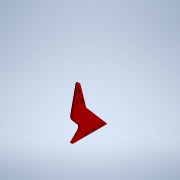
# Autodesk Inventor part: WeaponMountBasePlateV2
Saved by Autodesk Inventor 2020 (Build 240168000, 168)
## iProperties
Created: 2024-02-06
Part Number: WeaponMountBasePlateV2
Material: PETG
Document SubType Name: Modeling
Designer: smz3rm
Density: 1 g/cm^3
Appearance: Generic
Mass: 9.49681 g
Surface Area: 76.5782 cm^2
Volume: 9.49681 cm^3
WeaponHeight: 50.450 mm
SlotWidth: 6.000 mm
WeaponBite: 30.000 mm
WeaponMotorDia: 27.800 mm
SlotSpacing: 16.333 mm
SlotOffset: 2.000 mm
SlotHeight: 4.000 mm
SlotTolerance: 0.800 mm
WeaponMountBaseThinThickness: 1.000 mm
Height: 30.000 mm
BaseThickness: 3.000 mm
SideThickness: 6.000 mm
TopThickness: 1.000 mm
M3ScrewInsertBrim: 8.000 mm
M3ScrewDia: 3.100 mm
M3ScrewInsertDia: 4.000 mm
VM3ScrewInsertDia: 3.750 mm
FrontAngle: 45.00 deg
WeaponOpeningWidth: 15.000 mm
WeaponAssemblyWidth: 35.000 mm
WeaponCenterToMotorBack: 32.000 mm
WeaponMountThickness: 5.000 mm
WeaponDia: 88.900 mm
WeaponThickness: 3.000 mm
WeaponClearance: 10.000 mm
WeaponMotorShaftDia: 4.500 mm
WeaponMountWidth: 55.000 mm
Author: smz3rm
Autodesk Inventor part; units mm, degrees
ref_plane "YZ Plane" through (0, 0, 0) normal (1, 0, 0) x (0, 1, 0)
ref_plane "XZ Plane" through (0, 0, 0) normal (0, 1, 0) x (-1, 0, 0)
ref_plane "XY Plane" through (0, 0, 0) normal (0, 0, 1) x (1, 0, 0)
sketch "Sketch1" plane through (0, 0, 0) normal (1, 0, 0) x (0, 1, 0)
  line L0 (0, 0) -> (27, -27)
  line L1 (27, -27) -> (0, -27)
  line L2 (0, -27) -> (0, 0)
  line L3 (0, -76) -> (0, -27)
  arc A0 (53.3602, -0.8581) -> (59.496, -25.0037) centre (50.45, -14.45) ccw
  line L4 (6.4, -27) -> (1.6, -27)
  line L5 (1.6, -27) -> (1.6, -33.8)
  line L6 (1.6, -33.8) -> (6.4, -33.8)
  line L7 (6.4, -33.8) -> (6.4, -27)
  line L8 (1.6, -50.1333) -> (6.4, -50.1333)
  line L9 (6.4, -43.3333) -> (1.6, -43.3333)
  line L10 (1.6, -43.3333) -> (1.6, -50.1333)
  line L11 (6.4, -50.1333) -> (6.4, -43.3333)
  line L12 (1.6, -66.4667) -> (6.4, -66.4667)
  line L13 (6.4, -59.6667) -> (1.6, -59.6667)
  line L14 (1.6, -59.6667) -> (1.6, -66.4667)
  line L15 (6.4, -66.4667) -> (6.4, -59.6667)
  line L16 (0, -76) -> (59.496, -25.0037)
  arc A1 (105.5083, -16.8749) -> (105.4234, -12.0054) centre (104.9, -14.45) ccw
  line L17 (53.3602, -0.8581) -> (105.4234, -12.0054)
  line L18 (53.8652, -29.83) -> (105.5083, -16.8749)
  arc A2 (59.496, -25.0037) -> (53.3602, -0.8581) centre (50.45, -14.45) ccw
  line L19 (65.361, -6.4956) -> (102.6916, -14.4885)
  line L20 (102.6916, -14.4885) -> (64.3127, -24.1162)
  line L21 (21.2075, -21.2075) -> (41.404, -3.8963)
  line L22 (27, -27) -> (21.2075, -21.2075)
  circle A3 centre (10, -30) radius 1.55
  circle A4 centre (10, -56) radius 1.55
  arc A5 (64.3127, -24.1162) -> (65.361, -6.4956) centre (50.45, -14.45) ccw
  point P0 (0, -25.1779)
  point P1 (1.6, -27)
  dimension "SlotWidth" = 6
  dimension "SlotSpacing" = 16.3333
  dimension "SlotTolerance" = 0.8
  dimension "d0" = 45
  dimension "d1" = 27
  dimension "d34" = 27.8
  dimension "d40" = 50.45
  dimension "d55" = 4.8
  dimension "d56" = 6.8
  dimension "d57" = 1.6
  dimension "d60" = 16.3333
  dimension "d65" = 5
  dimension "d66" = 14.45
  dimension "d67" = 104.9
  dimension "d72" = 3
  dimension "d81" = 49
  dimension "d100" = 14.45
  dimension "d102" = 76
  dimension "d103" = 3.1
  dimension "d104" = 10
  dimension "d105" = 30
  dimension "d106" = 3.1
  dimension "d108" = 56
  dimension "d109" = 10
  dimension "d110" = 3
  constraints: 46 end point, 9 point on circle, 6 centre point, 5 tangent, 3 parallel, 3 point on line, 2 horizontal, 2 perpendicular, 2 vertical, 1 coincident, 1 collinear, 1 equal length, 17 other
  measures "d0" angle of L2 L0
  measures "d1" distance of L0.end L1.end
  measures "d34" diameter of A0
  measures "d40" distance from line of L3 point (50.45, -14.45)
  measures "d55" distance of L6.end L5.end
  measures "d56" distance of L5.end L4.end
  measures "d57" distance between parallel lines of L3 L5
  measures "d60" distance of L5.end L8.start
  measures "d65" diameter of A1
  measures "d66" vertical distance of L0.start A1.centre
  measures "d67" distance from line of L3 A1.centre
  measures "d72" distance between parallel lines of L17 L19
  measures "d81" distance from line of L3.start L1
  measures "d100" vertical distance of point (50.45, -14.45) L0.start
  measures "d102" distance of L3.start L0.start
  measures "d103" diameter of A3
  measures "d104" distance from line of L2 A3.centre
  measures "d105" vertical distance of L0.start A3.centre
  measures "d106" diameter of A4
  measures "d108" vertical distance of L0.start A4.centre
  measures "d109" distance from line of L3 A4.centre
  measures "d110" radial gap between concentric circles of A2 A5
extrude "Extrusion1" add sketch "Sketch1" along normal blind 5 contours L0 L1 L2 | L21 A0 L16 L3 L1 L5 L6 L7 L0 | A0 A2 | L17 A1 L18 L16 A2
sketch "Sketch9" plane through (5, 0, 0) normal (1, 0, 0) x (0, 0, -1)
  line L0 (6.4956, 65.361) -> (14.4885, 102.6916) projected
  arc A0 (24.1162, 64.3127) -> (6.4956, 65.361) centre (14.45, 50.45) ccw projected
  line L1 (14.4885, 102.6916) -> (24.1162, 64.3127) projected
  line L2 (6.4956, 65.361) -> (14.4885, 102.6916) projected
  line L3 (10.492, 84.0263) -> (19.3024, 83.5022)
  line L4 (15.4536, 67.3202) -> (10.492, 84.0263)
  line L5 (19.3024, 83.5022) -> (15.4536, 67.3202)
  line L6 (10.8097, 85.5101) -> (18.9197, 85.0276)
  line L7 (10.1743, 82.5425) -> (19.8519, 81.9668)
  line L8 (6.4956, 65.361) -> (14.4885, 102.6916) projected
  line L9 (9.8365, 80.9648) -> (13.8828, 67.3405)
  arc A1 (24.1162, 64.3127) -> (6.4956, 65.361) centre (14.45, 50.45) ccw projected
  line L10 (20.0938, 80.3472) -> (16.9581, 67.1629)
  line L11 (11.1475, 87.0878) -> (17.0702, 67.1456)
  arc A2 (24.1162, 64.3127) -> (6.4956, 65.361) centre (14.45, 50.45) ccw projected
  line L12 (13.9169, 67.3416) -> (18.5109, 86.6572)
  point P0 (17.4296, 82.1109)
  point P1 (15.2933, 73.1287)
  point P2 (12.5392, 82.4019)
  dimension "d111" = 3
  dimension "d112" = 1.5
  dimension "d113" = 3
  dimension "d114" = 3
  dimension "d115" = 1.5
  dimension "d116" = 1.5
  constraints: 18 end point, 7 point on line, 6 parallel, 5 point on circle, 2 midpoint
  measures "d111" distance between parallel lines of L7 L6
  measures "d112" distance between parallel lines of L6 L3
  measures "d113" distance between parallel lines of L11 L9
  measures "d114" distance between parallel lines of L10 L12
  measures "d115" distance between parallel lines of L4 L9
  measures "d116" distance between parallel lines of L10 L5
extrude "Extrusion9" add sketch "Sketch9" against normal up to surface (5 mm away) contours L0 L7 L4 L12 A0 L9 | L0 L4 L7 | L12 L4 A0 | L0 L6 L11 L3 | L3 L11 L7 L4 | L7 L11 L12 L4 | L5 L11 L10 A0 | L4 L12 L11 L5 | L11 L6 L12 L3 | L3 L12 L7 L11 | L11 L12 L7 L5 | L5 L7 L1 L10 L11 | L12 L6 L1 L3 | L3 L5 L7 L12 | L5 L1 L7
fillet "Fillet2" radius 10 2 edges at (2.5, 53.8652, -29.83) (2.5, 21.2075, -21.2075)
sketch "Sketch7" plane through (5, 0, 0) normal (1, 0, 0) x (0, 0, -1)
  arc A0 (16.8749, 105.5083) -> (12.0054, 105.4234) centre (14.45, 104.9) ccw projected
  line L0 (12.0054, 105.4234) -> (0.8581, 53.3602) projected
  arc A1 (0.8581, 53.3602) -> (3.8963, 41.404) centre (14.45, 50.45) ccw projected
  line L1 (3.8963, 41.404) -> (15.181, 28.2385) projected
  line L2 (76, 0) -> (31.3635, 52.0761) projected
  line L3 (29.2567, 56.1508) -> (16.8749, 105.5083) projected
  line L4 (66.4667, 1.6) -> (59.6667, 1.6) projected
  line L5 (27, 6.4) -> (33.8, 6.4) projected
  line L6 (27, 1.6) -> (27, 6.4) projected
  arc A2 (29.2567, 56.1508) -> (31.3635, 52.0761) centre (38.9561, 58.584) ccw projected
  arc A3 (14.6595, 14.6595) -> (15.181, 28.2385) centre (7.5884, 21.7306) ccw projected
  line L7 (33.8, 6.4) -> (33.8, 1.6) projected
  line L8 (33.8, 1.6) -> (27, 1.6) projected
  line L9 (66.4667, 6.4) -> (66.4667, 1.6) projected
  line L10 (59.6667, 1.6) -> (59.6667, 6.4) projected
  line L11 (59.6667, 6.4) -> (66.4667, 6.4) projected
  line L12 (14.6595, 14.6595) -> (0, 0) projected
  line L13 (0, 0) -> (76, 0) projected
  arc A4 (13.8828, 67.3405) -> (6.4956, 65.361) centre (14.45, 50.45) ccw projected
  line L14 (10.8097, 85.5101) -> (14.4885, 102.6916) projected
  line L15 (20.0938, 80.3472) -> (24.1162, 64.3127) projected
  line L16 (6.4956, 65.361) -> (9.8365, 80.9648) projected
  line L17 (9.8365, 80.9648) -> (13.8828, 67.3405) projected
  line L18 (16.9581, 67.1629) -> (20.0938, 80.3472) projected
  arc A5 (24.1162, 64.3127) -> (16.9581, 67.1629) centre (14.45, 50.45) ccw projected
  line L19 (18.9197, 85.0276) -> (10.8097, 85.5101) projected
  line L20 (14.4885, 102.6916) -> (18.9197, 85.0276) projected
  point P0 (23.7912, 23.7912)
  point P1 (17.4514, 17.4514)
fillet "Fillet3" radius 0.5 24 edges at (5, 6.4, -30.4) (5, 4, -27) (5, 1.6, -30.4) (0, 4, -27) (0, 6.4, -30.4) (0, 1.6, -30.4) (5, 4, -33.8) (0, 4, -33.8) (5, 4, -43.3333) (0, 4, -43.3333) (5, 1.6, -46.7333) (5, 6.4, -46.7333) (0, 4, -50.1333) (5, 4, -50.1333) (5, 4, -59.6667) (5, 6.4, -63.0667) (5, 1.6, -63.0667) (5, 4, -66.4667) (0, 4, -66.4667) (0, 4, -59.6667) (0, 1.6, -63.0667) (0, 6.4, -63.0667) (0, 1.6, -46.7333) (0, 6.4, -46.7333)
sketch "Sketch8" plane through (5, 0, 0) normal (1, 0, 0) x (0, 0, -1)
  circle A0 centre (20, 12) radius 1.8
  point P0 (0, 0)
  dimension "d76" = 3.6
  dimension "d77" = 12
  dimension "d78" = 20
  constraints: 1 centre point
  measures "d76" diameter of A0
  measures "d77" vertical distance of point (0, 0) A0.centre
  measures "d78" horizontal distance of A0.centre point (0, 0)
extrude "Extrusion8" cut sketch "Sketch8" against normal through all
fillet "Fillet4" radius 1.5 2 edges at (2.5, 65.361, -6.4956) (2.5, 64.3127, -24.1162)
fillet "Fillet5" radius 1 10 edges at (2.5, 85.5101, -10.8097) (2.5, 85.0276, -18.9197) (2.5, 82.4019, -12.5392) (2.5, 82.1109, -17.4296) (2.5, 73.1287, -15.2933) (2.5, 67.3405, -13.8828) (2.5, 80.9648, -9.8365) (2.5, 80.3472, -20.0938) (2.5, 67.1629, -16.9581) (2.5, 102.6916, -14.4885)
equation "\"SlotWidth\" = 6"
equation "\"SlotSpacing\" = 16.33333"
equation "\"SlotTolerance\" = 0.8"
equation "\"d0\" = FrontAngle"
equation "\"d1\" = Height - BaseThickness"
equation "\"d34\" = WeaponMotorDia"
equation "\"WeaponHeight\" = 50.45"
equation "\"WeaponBite\" = 30"
equation "\"WeaponMotorDia\" = 27.8"
equation "\"SlotOffset\" = 2"
equation "\"SlotHeight\" = 4"
equation "\"WeaponMountBaseThinThickness\" = 1"
equation "\"WeaponBodyOffset\" = 77.9"
equation "\"WeaponLengthOffset\" = 162.55"
equation "\"BumpLengthOffset\" = 162.55"
equation "\"BumpHeight\" = 104.9"
equation "\"WeaponMountRearAngle\" = 50deg"
equation "\"FrontAngle\" = 45deg"
equation "\"Height\" = 30"
equation "\"BaseThickness\" = 3"
body "Solid1"
